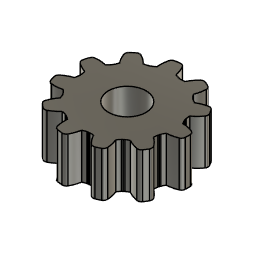
Pinion v6 (Autodesk Fusion 360 design; units mm, degrees)
Autodesk Fusion 360 part; units mm, degrees
(part 1 of 2)
sketch "Sketch1" plane through (0, 0, 0) normal (0, 0, 1) x (1, 0, 0)
sketch "Sketch2" plane through (0, 0, 0) normal (0, 0, 1) x (1, 0, 0)
  circle A0 centre (-2.1465, 3.0724) radius 9.2859
  spline S0 degree 5 poles (-1.9793, 9.7968) (-1.9628, 9.789) (-1.9296, 9.7738) (-1.8797, 9.7518) (-1.813, 9.7244) (-1.7292, 9.6933) (-1.6451, 9.6655) (-1.5605, 9.6411) (-1.4754, 9.6201) (-1.3897, 9.6025) (-1.3033, 9.5881) (-1.2161, 9.5769) (-1.128, 9.5685) (-1.039, 9.563) (-0.949, 9.5599) (-0.8581, 9.5593) (-0.7846, 9.5607) (-0.7291, 9.5627) (-0.6919, 9.5645) (-0.6732, 9.5655) knots 0 0 0 0 0 0 0.066667 0.133333 0.2 0.266667 0.333333 0.4 0.466667 0.533333 0.6 0.666667 0.733333 0.8 0.866667 0.933333 1 1 1 1 1 1
  line L0 (-2.6468, 6.3471) -> (-2.1465, 3.0724)
  spline S1 degree 5 poles (-4.3138, 9.4402) (-4.3273, 9.4278) (-4.3544, 9.4033) (-4.3954, 9.3675) (-4.4509, 9.3214) (-4.5216, 9.2667) (-4.5936, 9.2151) (-4.6671, 9.1665) (-4.742, 9.1211) (-4.8185, 9.0787) (-4.8967, 9.0392) (-4.9765, 9.0024) (-5.0581, 8.9682) (-5.1414, 8.9362) (-5.2264, 8.9065) (-5.313, 8.8788) (-5.3835, 8.8581) (-5.4371, 8.8435) (-5.4732, 8.8341) (-5.4913, 8.8295) knots 0 0 0 0 0 0 0.066667 0.133333 0.2 0.266667 0.333333 0.4 0.466667 0.533333 0.6 0.666667 0.733333 0.8 0.866667 0.933333 1 1 1 1 1 1
  line L1 (-2.1078, 9.8571) -> (-1.8509, 9.7365)
  line L2 (-0.8154, 9.5579) -> (-0.5311, 9.5732)
  line L3 (-4.2092, 9.5361) -> (-4.4184, 9.3442)
  line L4 (-5.3533, 8.8646) -> (-5.6292, 8.7944)
  arc A1 (-1.9793, 9.7968) -> (-3.3455, 12.2806) centre (-6.5618, 8.894) ccw
  arc A2 (-3.7515, 12.2186) -> (-4.3138, 9.4402) centre (0.3292, 9.9467) ccw
  arc A3 (-8.4415, 9.8989) -> (-7.4124, 7.2576) centre (-3.7804, 10.1939) ccw
  arc A4 (-5.6414, 8.8197) -> (-8.1335, 10.1706) centre (-9.0082, 5.5828) ccw
  spline S2 degree 5 poles (-5.6414, 8.8197) (-5.6232, 8.8221) (-5.587, 8.8272) (-5.5332, 8.8357) (-5.4623, 8.8487) (-5.375, 8.8679) (-5.2892, 8.89) (-5.2048, 8.9152) (-5.1219, 8.9435) (-5.0403, 8.9751) (-4.9598, 9.0097) (-4.8804, 9.0473) (-4.8018, 9.0879) (-4.7239, 9.1314) (-4.6466, 9.1775) (-4.5697, 9.2261) (-4.5086, 9.267) (-4.463, 9.2987) (-4.4327, 9.3204) (-4.4176, 9.3313) knots 0 0 0 0 0 0 0.066667 0.133333 0.2 0.266667 0.333333 0.4 0.466667 0.533333 0.6 0.666667 0.733333 0.8 0.866667 0.933333 1 1 1 1 1 1
  spline S3 degree 5 poles (-7.4124, 7.2576) (-7.4171, 7.2399) (-7.4267, 7.2046) (-7.4418, 7.1523) (-7.4636, 7.0835) (-7.4935, 6.9993) (-7.5261, 6.9169) (-7.5617, 6.8364) (-7.6001, 6.7576) (-7.6416, 6.6806) (-7.686, 6.6051) (-7.7333, 6.531) (-7.7834, 6.4581) (-7.8362, 6.3862) (-7.8916, 6.3153) (-7.9495, 6.2451) (-7.9977, 6.1896) (-8.0348, 6.1483) (-8.0601, 6.1209) (-8.0728, 6.1073) knots 0 0 0 0 0 0 0.066667 0.133333 0.2 0.266667 0.333333 0.4 0.466667 0.533333 0.6 0.666667 0.733333 0.8 0.866667 0.933333 1 1 1 1 1 1
  arc A5 (-11.1329, 5.4119) -> (-8.8391, 3.7463) centre (-7.3712, 8.1801) ccw
  arc A6 (-8.1938, 6.0179) -> (-11.0207, 5.807) centre (-9.2762, 1.4745) ccw
  spline S4 degree 5 poles (-8.1938, 6.0179) (-8.1798, 6.0297) (-8.1522, 6.0536) (-8.1115, 6.0898) (-8.0588, 6.1391) (-7.9958, 6.2024) (-7.9355, 6.2674) (-7.8782, 6.3342) (-7.8237, 6.4029) (-7.7721, 6.4735) (-7.7232, 6.5462) (-7.6767, 6.6208) (-7.6325, 6.6975) (-7.5905, 6.7761) (-7.5503, 6.8567) (-7.512, 6.9392) (-7.4827, 7.0066) (-7.4615, 7.0579) (-7.4477, 7.0925) (-7.4409, 7.1099) knots 0 0 0 0 0 0 0.066667 0.133333 0.2 0.266667 0.333333 0.4 0.466667 0.533333 0.6 0.666667 0.733333 0.8 0.866667 0.933333 1 1 1 1 1 1
  spline S5 degree 5 poles (-8.8391, 3.7463) (-8.8335, 3.7288) (-8.8225, 3.694) (-8.807, 3.6418) (-8.7881, 3.5722) (-8.7677, 3.4852) (-8.7506, 3.3982) (-8.737, 3.3112) (-8.7268, 3.2242) (-8.72, 3.137) (-8.7166, 3.0494) (-8.7163, 2.9615) (-8.719, 2.8731) (-8.7246, 2.7841) (-8.7328, 2.6944) (-8.7436, 2.6041) (-8.7541, 2.5314) (-8.7631, 2.4766) (-8.7695, 2.4399) (-8.7728, 2.4215) knots 0 0 0 0 0 0 0.066667 0.133333 0.2 0.266667 0.333333 0.4 0.466667 0.533333 0.6 0.666667 0.733333 0.8 0.866667 0.933333 1 1 1 1 1 1
  arc A7 (-10.9712, 0.1821) -> (-8.141, 0.021) centre (-9.3032, 4.5446) ccw
  arc A8 (-8.8263, 2.2809) -> (-11.0904, 0.5752) centre (-7.2805, -2.1264) ccw
  spline S6 degree 5 poles (-8.8263, 2.2809) (-8.8209, 2.2984) (-8.8105, 2.3334) (-8.7959, 2.3859) (-8.7783, 2.4559) (-8.7594, 2.5432) (-8.7439, 2.6305) (-8.7318, 2.7177) (-8.7231, 2.8049) (-8.7179, 2.8922) (-8.716, 2.9798) (-8.7172, 3.0677) (-8.7215, 3.156) (-8.7286, 3.2449) (-8.7384, 3.3344) (-8.7508, 3.4245) (-8.7626, 3.4971) (-8.7725, 3.5517) (-8.7796, 3.5883) (-8.7832, 3.6066) knots 0 0 0 0 0 0 0.066667 0.133333 0.2 0.266667 0.333333 0.4 0.466667 0.533333 0.6 0.666667 0.733333 0.8 0.866667 0.933333 1 1 1 1 1 1
  spline S7 degree 5 poles (-8.141, 0.021) (-8.1269, 0.0094) (-8.0988, -0.014) (-8.0575, -0.0495) (-8.004, -0.0979) (-7.9398, -0.16) (-7.8784, -0.224) (-7.8199, -0.2898) (-7.7643, -0.3575) (-7.7114, -0.4272) (-7.6612, -0.4989) (-7.6134, -0.5727) (-7.5679, -0.6486) (-7.5245, -0.7265) (-7.4829, -0.8064) (-7.4432, -0.8882) (-7.4127, -0.9551) (-7.3906, -1.006) (-7.3762, -1.0404) (-7.369, -1.0576) knots 0 0 0 0 0 0 0.066667 0.133333 0.2 0.266667 0.333333 0.4 0.466667 0.533333 0.6 0.666667 0.733333 0.8 0.866667 0.933333 1 1 1 1 1 1
  arc A9 (-8.0077, -4.1301) -> (-5.5397, -2.7355) centre (-8.963, 0.4417) ccw
  arc A10 (-7.338, -1.2048) -> (-8.3205, -3.8638) centre (-3.6548, -4.0767) ccw
  spline S8 degree 5 poles (-7.338, -1.2048) (-7.3429, -1.1872) (-7.3531, -1.1521) (-7.3692, -1.1) (-7.3922, -1.0316) (-7.4235, -0.948) (-7.4576, -0.8662) (-7.4946, -0.7863) (-7.5345, -0.7082) (-7.5773, -0.6319) (-7.623, -0.5572) (-7.6716, -0.484) (-7.723, -0.4119) (-7.777, -0.341) (-7.8337, -0.271) (-7.8928, -0.2019) (-7.9419, -0.1473) (-7.9798, -0.1066) (-8.0055, -0.0797) (-8.0185, -0.0663) knots 0 0 0 0 0 0 0.066667 0.133333 0.2 0.266667 0.333333 0.4 0.466667 0.533333 0.6 0.666667 0.733333 0.8 0.866667 0.933333 1 1 1 1 1 1
  spline S9 degree 5 poles (-5.5397, -2.7355) (-5.5215, -2.7376) (-5.4853, -2.7421) (-5.4313, -2.7496) (-5.3601, -2.7614) (-5.2725, -2.779) (-5.1863, -2.7996) (-5.1015, -2.8233) (-5.0181, -2.8502) (-4.936, -2.8803) (-4.8549, -2.9135) (-4.7749, -2.9497) (-4.6955, -2.9889) (-4.6169, -3.031) (-4.5388, -3.0757) (-4.4611, -3.123) (-4.3993, -3.1628) (-4.3531, -3.1937) (-4.3224, -3.2148) (-4.3071, -3.2255) knots 0 0 0 0 0 0 0.066667 0.133333 0.2 0.266667 0.333333 0.4 0.466667 0.533333 0.6 0.666667 0.733333 0.8 0.866667 0.933333 1 1 1 1 1 1
  arc A11 (-3.1833, -6.1555) -> (-1.8611, -3.648) centre (-6.4587, -2.826) ccw
  arc A12 (-4.2014, -3.3325) -> (-3.5904, -6.1006) centre (0.4497, -3.7573) ccw
  spline S10 degree 5 poles (-4.2014, -3.3325) (-4.2151, -3.3204) (-4.2427, -3.2964) (-4.2843, -3.2613) (-4.3406, -3.2162) (-4.4122, -3.1627) (-4.4852, -3.1124) (-4.5594, -3.0651) (-4.6352, -3.021) (-4.7124, -2.98) (-4.7913, -2.9419) (-4.8718, -2.9065) (-4.9539, -2.8737) (-5.0378, -2.8432) (-5.1233, -2.815) (-5.2103, -2.7888) (-5.2812, -2.7694) (-5.3351, -2.7557) (-5.3713, -2.7469) (-5.3895, -2.7427) knots 0 0 0 0 0 0 0.066667 0.133333 0.2 0.266667 0.333333 0.4 0.466667 0.533333 0.6 0.666667 0.733333 0.8 0.866667 0.933333 1 1 1 1 1 1
  spline S11 degree 5 poles (-1.8611, -3.648) (-1.8446, -3.6399) (-1.8117, -3.6241) (-1.7622, -3.6013) (-1.696, -3.5727) (-1.6128, -3.5401) (-1.5292, -3.5109) (-1.445, -3.485) (-1.3603, -3.4625) (-1.2749, -3.4434) (-1.1888, -3.4275) (-1.1018, -3.4147) (-1.0139, -3.4048) (-0.925, -3.3977) (-0.8351, -3.3931) (-0.7442, -3.3909) (-0.6707, -3.3909) (-0.6151, -3.392) (-0.5779, -3.3931) (-0.5592, -3.3938) knots 0 0 0 0 0 0 0.066667 0.133333 0.2 0.266667 0.333333 0.4 0.466667 0.533333 0.6 0.666667 0.733333 0.8 0.866667 0.933333 1 1 1 1 1 1
  arc A13 (1.9703, -5.2511) -> (1.727, -2.4268) centre (-2.5852, -4.2209) ccw
  arc A14 (-0.4125, -3.4267) -> (1.5981, -5.425) centre (3.73, -1.2694) ccw
  spline S12 degree 5 poles (-0.4125, -3.4267) (-0.4306, -3.4239) (-0.4667, -3.4186) (-0.5207, -3.4116) (-0.5925, -3.4041) (-0.6816, -3.3979) (-0.7702, -3.3949) (-0.8582, -3.3953) (-0.9458, -3.3992) (-1.033, -3.4064) (-1.1199, -3.417) (-1.2067, -3.4307) (-1.2936, -3.4476) (-1.3806, -3.4673) (-1.4678, -3.4897) (-1.5552, -3.5148) (-1.6253, -3.5368) (-1.678, -3.5544) (-1.7132, -3.5666) (-1.7308, -3.5728) knots 0 0 0 0 0 0 0.066667 0.133333 0.2 0.266667 0.333333 0.4 0.466667 0.533333 0.6 0.666667 0.733333 0.8 0.866667 0.933333 1 1 1 1 1 1
  spline S13 degree 5 poles (1.727, -2.4268) (1.7364, -2.4112) (1.7555, -2.38) (1.7848, -2.3341) (1.8251, -2.2742) (1.8775, -2.2019) (1.932, -2.132) (1.9888, -2.0647) (2.0479, -2) (2.1094, -1.9378) (2.1733, -1.8779) (2.2395, -1.8201) (2.3082, -1.7642) (2.3791, -1.7102) (2.4522, -1.6577) (2.5275, -1.6067) (2.5894, -1.567) (2.6367, -1.5379) (2.6686, -1.5187) (2.6847, -1.5092) knots 0 0 0 0 0 0 0.066667 0.133333 0.2 0.266667 0.333333 0.4 0.466667 0.533333 0.6 0.666667 0.733333 0.8 0.866667 0.933333 1 1 1 1 1 1
  arc A15 (5.8168, -1.7041) -> (4.0852, 0.5403) centre (1.4275, -3.3003) ccw
  arc A16 (2.8259, -1.4575) -> (5.5977, -2.0516) centre (5.1445, 2.5969) ccw
  spline S14 degree 5 poles (2.8259, -1.4575) (2.8092, -1.4649) (2.776, -1.48) (2.7267, -1.5033) (2.6623, -1.5358) (2.5839, -1.5787) (2.5078, -1.6241) (2.434, -1.6721) (2.3624, -1.7227) (2.293, -1.7759) (2.2256, -1.8318) (2.1599, -1.8903) (2.096, -1.9514) (2.0334, -2.015) (1.9722, -2.081) (1.9122, -2.1494) (1.8651, -2.2058) (1.8303, -2.2491) (1.8073, -2.2784) (1.7959, -2.2931) knots 0 0 0 0 0 0 0.066667 0.133333 0.2 0.266667 0.333333 0.4 0.466667 0.533333 0.6 0.666667 0.733333 0.8 0.866667 0.933333 1 1 1 1 1 1
  spline S15 degree 5 poles (4.0852, 0.5403) (4.0846, 0.5586) (4.0839, 0.5951) (4.0837, 0.6496) (4.0852, 0.7217) (4.0902, 0.8109) (4.0983, 0.8992) (4.1097, 0.9865) (4.1244, 1.0729) (4.1425, 1.1585) (4.1639, 1.2434) (4.1883, 1.3279) (4.2159, 1.4119) (4.2463, 1.4958) (4.2795, 1.5795) (4.3152, 1.6631) (4.3458, 1.7299) (4.3699, 1.78) (4.3864, 1.8134) (4.3947, 1.8301) knots 0 0 0 0 0 0 0.066667 0.133333 0.2 0.266667 0.333333 0.4 0.466667 0.533333 0.6 0.666667 0.733333 0.8 0.866667 0.933333 1 1 1 1 1 1
  arc A17 (7.135, 3.3594) -> (4.4649, 4.3114) centre (4.3055, -0.3564) ccw
  arc A18 (4.4856, 1.9499) -> (7.1386, 2.9487) centre (4.2442, 6.6142) ccw
  spline S16 degree 5 poles (4.4856, 1.9499) (4.4756, 1.9346) (4.4557, 1.904) (4.4269, 1.8577) (4.3903, 1.7956) (4.3476, 1.7171) (4.3081, 1.6378) (4.2719, 1.5575) (4.239, 1.4762) (4.2094, 1.3939) (4.1829, 1.3105) (4.1593, 1.2258) (4.1386, 1.1398) (4.1204, 1.0525) (4.1046, 0.9638) (4.091, 0.8739) (4.0819, 0.801) (4.076, 0.7457) (4.0725, 0.7086) (4.0709, 0.69) knots 0 0 0 0 0 0 0.066667 0.133333 0.2 0.266667 0.333333 0.4 0.466667 0.533333 0.6 0.666667 0.733333 0.8 0.866667 0.933333 1 1 1 1 1 1
  spline S17 degree 5 poles (4.4649, 4.3114) (4.4545, 4.3265) (4.4342, 4.3568) (4.4045, 4.4026) (4.3668, 4.464) (4.3228, 4.5418) (4.2819, 4.6204) (4.2443, 4.7) (4.21, 4.7806) (4.1789, 4.8624) (4.1509, 4.9454) (4.1259, 5.0297) (4.1036, 5.1153) (4.0838, 5.2023) (4.0665, 5.2906) (4.0514, 5.3803) (4.041, 5.4531) (4.0341, 5.5082) (4.03, 5.5452) (4.028, 5.5638) knots 0 0 0 0 0 0 0.066667 0.133333 0.2 0.266667 0.333333 0.4 0.466667 0.533333 0.6 0.666667 0.733333 0.8 0.866667 0.933333 1 1 1 1 1 1
  arc A19 (5.5064, 8.3318) -> (2.7455, 7.6891) centre (5.135, 3.6761) ccw
  arc A20 (4.0396, 5.7137) -> (5.7315, 7.9882) centre (1.3148, 9.507) ccw
  spline S18 degree 5 poles (4.0396, 5.7137) (4.0395, 5.6954) (4.0394, 5.6589) (4.0401, 5.6044) (4.0429, 5.5323) (4.0494, 5.4432) (4.0591, 5.3551) (4.072, 5.268) (4.0883, 5.1819) (4.1079, 5.0967) (4.1307, 5.0121) (4.1567, 4.9281) (4.1857, 4.8445) (4.2176, 4.7612) (4.2522, 4.6781) (4.2894, 4.5952) (4.3212, 4.5289) (4.3461, 4.4792) (4.3632, 4.4461) (4.3719, 4.4296) knots 0 0 0 0 0 0 0.066667 0.133333 0.2 0.266667 0.333333 0.4 0.466667 0.533333 0.6 0.666667 0.733333 0.8 0.866667 0.933333 1 1 1 1 1 1
  spline S19 degree 5 poles (2.7455, 7.6891) (2.7286, 7.6962) (2.6951, 7.7107) (2.6454, 7.7332) (2.5805, 7.7645) (2.5014, 7.8061) (2.4245, 7.8501) (2.3498, 7.8967) (2.2773, 7.946) (2.207, 7.998) (2.1386, 8.0527) (2.072, 8.1101) (2.0069, 8.1701) (1.9433, 8.2326) (1.8809, 8.2975) (1.8197, 8.3648) (1.7717, 8.4204) (1.7361, 8.463) (1.7126, 8.4919) (1.7009, 8.5065) knots 0 0 0 0 0 0 0.066667 0.133333 0.2 0.266667 0.333333 0.4 0.466667 0.533333 0.6 0.666667 0.733333 0.8 0.866667 0.933333 1 1 1 1 1 1
  arc A21 (1.4481, 11.6344) -> (-0.5271, 9.601) centre (3.6527, 7.517) ccw
  arc A22 (1.6296, 8.6389) -> (1.8232, 11.467) centre (-2.7135, 10.3569) ccw
  spline S20 degree 5 poles (1.6296, 8.6389) (1.6393, 8.6234) (1.659, 8.5926) (1.6891, 8.5472) (1.7304, 8.4881) (1.7841, 8.4166) (1.8398, 8.3478) (1.8978, 8.2815) (1.958, 8.2178) (2.0206, 8.1567) (2.0855, 8.0979) (2.1528, 8.0413) (2.2224, 7.9867) (2.2942, 7.9338) (2.3683, 7.8826) (2.4445, 7.833) (2.507, 7.7944) (2.5548, 7.7661) (2.5871, 7.7475) (2.6033, 7.7383) knots 0 0 0 0 0 0 0.066667 0.133333 0.2 0.266667 0.333333 0.4 0.466667 0.533333 0.6 0.666667 0.733333 0.8 0.866667 0.933333 1 1 1 1 1 1
  spline S21 degree 5 poles (-0.5271, 9.601) (-0.5451, 9.5979) (-0.5812, 9.592) (-0.6351, 9.584) (-0.7067, 9.5752) (-0.7957, 9.5674) (-0.8842, 9.5629) (-0.9722, 9.5618) (-1.0598, 9.5641) (-1.1471, 9.5698) (-1.2342, 9.5788) (-1.3213, 9.5911) (-1.4084, 9.6063) (-1.4957, 9.6245) (-1.5833, 9.6454) (-1.6712, 9.669) (-1.7417, 9.6897) (-1.7947, 9.7064) (-1.8301, 9.718) (-1.8478, 9.7239) knots 0 0 0 0 0 0 0.066667 0.133333 0.2 0.266667 0.333333 0.4 0.466667 0.533333 0.6 0.666667 0.733333 0.8 0.866667 0.933333 1 1 1 1 1 1
  point P0 (-1.5603, 9.642)
  point P1 (-1.1296, 9.5694)
  point P2 (-4.6674, 9.1673)
  point P3 (-5.0568, 8.9694)
  point P4 (-5.2052, 8.916)
  point P5 (-4.8036, 9.0878)
  point P6 (-7.5624, 6.8368)
  point P7 (-7.783, 6.4599)
  point P8 (-7.8789, 6.3347)
  point P9 (-7.6339, 6.6963)
  point P10 (-8.7378, 3.3112)
  point P11 (-8.7196, 2.8748)
  point P12 (-8.7326, 2.7177)
  point P13 (-8.7221, 3.1543)
  point P14 (-7.8206, -0.2903)
  point P15 (-7.5693, -0.6475)
  point P16 (-7.4953, -0.7867)
  point P17 (-7.7225, -0.4137)
  point P18 (-5.1019, -2.8241)
  point P19 (-4.6973, -2.9888)
  point P20 (-4.5598, -3.0659)
  point P21 (-4.9526, -2.8749)
  point P22 (-1.4448, -3.4858)
  point P23 (-1.0155, -3.4057)
  point P24 (-0.8581, -3.3962)
  point P25 (-1.2918, -3.4479)
  point P26 (1.9894, -2.0654)
  point P27 (2.3073, -1.7658)
  point P28 (2.4345, -1.6728)
  point P29 (2.0976, -1.9507)
  point P30 (4.1105, 0.9863)
  point P31 (4.216, 1.4101)
  point P32 (4.2727, 1.5572)
  point P33 (4.1396, 1.1412)
  point P34 (4.2451, 4.7003)
  point P35 (4.1047, 5.1139)
  point P36 (4.0729, 5.2683)
  point P37 (4.1858, 4.8463)
  point P38 (2.3504, 7.8974)
  point P39 (2.0086, 8.1694)
  point P40 (1.8984, 8.2821)
  point P41 (2.2215, 7.9882)
  point P42 (-0.9721, 9.5627)
  point P43 (-1.4067, 9.6067)
  dimension "d2" = 360
  constraint coincident A0.centre L0.end
  constraint midpoint S0.start L1
  constraint midpoint S0.end L2
  constraint symmetric S0.start L0 S1.start
  constraint symmetric P0 L0 P2
  constraint symmetric P1 L0 P3
  constraint symmetric S0.end L0 S1.end
  constraint symmetric L0 L1.start L3.start
  constraint symmetric L0 L1.end L3.end
  constraint symmetric L0 L2.start L4.start
  constraint symmetric L0 L2.end L4.end
  constraint coincident A0 A1.end
  constraint coincident A0 A2.start
  constraint coincident L0.start A2
extrude "Extrude1" add sketch "Sketch2" along normal blind 6.35 contours A0 S0 S1 A1 A2 A3 A4 S2 S3 A5 A6 S4 S5 A7 A8 S6 S7 A9 A10 S8 S9 A11 A12 S10 S11 A13 A14 S12 S13 A15 A16 S14 S15 A17 A18 S16 S17 A19 A20 S18 S19 A21 A22 S20 S21
sketch "Sketch3" plane through (0, 0, 6.35) normal (0, 0, 1) x (-1, 0, 0)
  arc A0 (-1.6296, -8.6389) -> (-1.8232, -11.467) centre (2.7135, -10.3569) ccw
  arc A1 (-1.8232, -11.467) -> (-1.4481, -11.6344) centre (2.1465, -3.0724) ccw
  arc A2 (-1.4481, -11.6344) -> (0.5271, -9.601) centre (-3.6527, -7.517) ccw
  spline S0 degree 5 poles (0.5271, -9.601) (0.5451, -9.5979) (0.5812, -9.592) (0.6351, -9.584) (0.7067, -9.5752) (0.7957, -9.5674) (0.8842, -9.5629) (0.9616, -9.5619) (1.0213, -9.5631) (1.0633, -9.565) (1.0877, -9.5664) (1.0947, -9.5668) knots 0 0 0 0 0 0 0.066667 0.133333 0.2 0.266667 0.333333 0.4 0.426673 0.426673 0.426673 0.426673 0.426673 0.426673
  spline S1 degree 5 poles (1.0947, -9.5668) (1.1052, -9.5675) (1.1331, -9.5693) (1.1679, -9.5722) (1.2027, -9.5757) (1.2375, -9.5799) (1.2618, -9.5831) (1.2687, -9.5841) knots 0.426673 0.426673 0.426673 0.426673 0.426673 0.426673 0.466667 0.533333 0.559717 0.559717 0.559717 0.559717 0.559717 0.559717
  spline S2 degree 5 poles (1.2687, -9.5841) (1.2756, -9.585) (1.2999, -9.5883) (1.3345, -9.5935) (1.369, -9.5993) (1.4033, -9.6058) (1.4307, -9.6113) (1.441, -9.6135) knots -0.559717 -0.559717 -0.559717 -0.559717 -0.559717 -0.559717 -0.533333 -0.466667 -0.426673 -0.426673 -0.426673 -0.426673 -0.426673 -0.426673
  spline S3 degree 5 poles (1.441, -9.6135) (1.4479, -9.6149) (1.4718, -9.6201) (1.5128, -9.6294) (1.5706, -9.644) (1.6451, -9.6655) (1.7292, -9.6933) (1.813, -9.7244) (1.8797, -9.7518) (1.9296, -9.7738) (1.9628, -9.789) (1.9793, -9.7968) knots -0.426673 -0.426673 -0.426673 -0.426673 -0.426673 -0.426673 -0.4 -0.333333 -0.266667 -0.2 -0.133333 -0.066667 0 0 0 0 0 0
  arc A3 (1.9793, -9.7968) -> (3.3455, -12.2806) centre (6.5618, -8.894) ccw
  arc A4 (3.3455, -12.2806) -> (3.7515, -12.2186) centre (2.1465, -3.0724) ccw
  arc A5 (3.7515, -12.2186) -> (4.3138, -9.4402) centre (-0.3292, -9.9467) ccw
  spline S4 degree 5 poles (4.3138, -9.4402) (4.3273, -9.4278) (4.3544, -9.4033) (4.3954, -9.3675) (4.4509, -9.3214) (4.5216, -9.2667) (4.5936, -9.2151) (4.6582, -9.1723) (4.7091, -9.1411) (4.7454, -9.12) (4.7667, -9.1079) (4.7728, -9.1045) knots 0 0 0 0 0 0 0.066667 0.133333 0.2 0.266667 0.333333 0.4 0.426673 0.426673 0.426673 0.426673 0.426673 0.426673
  spline S5 degree 5 poles (4.7728, -9.1045) (4.782, -9.0994) (4.8065, -9.0859) (4.8373, -9.0695) (4.8685, -9.0536) (4.9, -9.0383) (4.9222, -9.0279) (4.9285, -9.025) knots 0.426673 0.426673 0.426673 0.426673 0.426673 0.426673 0.466667 0.533333 0.559717 0.559717 0.559717 0.559717 0.559717 0.559717
  spline S6 degree 5 poles (4.9285, -9.025) (4.9348, -9.022) (4.9571, -9.0117) (4.989, -8.9973) (5.0211, -8.9836) (5.0535, -8.9704) (5.0796, -8.9603) (5.0894, -8.9566) knots -0.559717 -0.559717 -0.559717 -0.559717 -0.559717 -0.559717 -0.533333 -0.466667 -0.426673 -0.426673 -0.426673 -0.426673 -0.426673 -0.426673
  spline S7 degree 5 poles (5.0894, -8.9566) (5.0959, -8.9541) (5.1189, -8.9454) (5.1584, -8.9311) (5.2149, -8.9122) (5.2892, -8.89) (5.375, -8.8679) (5.4623, -8.8487) (5.5332, -8.8357) (5.587, -8.8272) (5.6232, -8.8221) (5.6414, -8.8197) knots -0.426673 -0.426673 -0.426673 -0.426673 -0.426673 -0.426673 -0.4 -0.333333 -0.266667 -0.2 -0.133333 -0.066667 0 0 0 0 0 0
  arc A6 (5.6414, -8.8197) -> (8.1335, -10.1706) centre (9.0082, -5.5828) ccw
  arc A7 (8.1335, -10.1706) -> (8.4415, -9.8989) centre (2.1465, -3.0724) ccw
  arc A8 (8.4415, -9.8989) -> (7.4124, -7.2576) centre (3.7804, -10.1939) ccw
  spline S8 degree 5 poles (7.4124, -7.2576) (7.4171, -7.2399) (7.4267, -7.2046) (7.4418, -7.1523) (7.4636, -7.0835) (7.4935, -6.9993) (7.5261, -6.9169) (7.5574, -6.8461) (7.5833, -6.7923) (7.6024, -6.7549) (7.6138, -6.7332) (7.6171, -6.727) knots 0 0 0 0 0 0 0.066667 0.133333 0.2 0.266667 0.333333 0.4 0.426673 0.426673 0.426673 0.426673 0.426673 0.426673
  spline S9 degree 5 poles (7.6171, -6.727) (7.6221, -6.7178) (7.6354, -6.6931) (7.6524, -6.6627) (7.6701, -6.6325) (7.6883, -6.6026) (7.7014, -6.5818) (7.7051, -6.576) knots 0.426673 0.426673 0.426673 0.426673 0.426673 0.426673 0.466667 0.533333 0.559717 0.559717 0.559717 0.559717 0.559717 0.559717
  spline S10 degree 5 poles (7.7051, -6.576) (7.7088, -6.5701) (7.7219, -6.5494) (7.741, -6.52) (7.7606, -6.4911) (7.7807, -6.4625) (7.7972, -6.4399) (7.8034, -6.4314) knots -0.559717 -0.559717 -0.559717 -0.559717 -0.559717 -0.559717 -0.533333 -0.466667 -0.426673 -0.426673 -0.426673 -0.426673 -0.426673 -0.426673
  spline S11 degree 5 poles (7.8034, -6.4314) (7.8076, -6.4258) (7.8222, -6.4061) (7.8477, -6.3727) (7.885, -6.3262) (7.9355, -6.2674) (7.9958, -6.2024) (8.0588, -6.1391) (8.1115, -6.0898) (8.1522, -6.0536) (8.1798, -6.0297) (8.1938, -6.0179) knots -0.426673 -0.426673 -0.426673 -0.426673 -0.426673 -0.426673 -0.4 -0.333333 -0.266667 -0.2 -0.133333 -0.066667 0 0 0 0 0 0
  arc A9 (8.1938, -6.0179) -> (11.0207, -5.807) centre (9.2762, -1.4745) ccw
  arc A10 (11.0207, -5.807) -> (11.1329, -5.4119) centre (2.1465, -3.0724) ccw
  arc A11 (11.1329, -5.4119) -> (8.8391, -3.7463) centre (7.3712, -8.1801) ccw
  spline S12 degree 5 poles (8.8391, -3.7463) (8.8335, -3.7288) (8.8225, -3.694) (8.807, -3.6418) (8.7881, -3.5722) (8.7677, -3.4852) (8.7506, -3.3982) (8.7386, -3.3217) (8.7313, -3.2625) (8.7272, -3.2207) (8.7251, -3.1962) (8.7245, -3.1893) knots 0 0 0 0 0 0 0.066667 0.133333 0.2 0.266667 0.333333 0.4 0.426673 0.426673 0.426673 0.426673 0.426673 0.426673
  spline S13 degree 5 poles (8.7245, -3.1893) (8.7237, -3.1788) (8.7216, -3.1509) (8.7194, -3.116) (8.718, -3.0811) (8.7172, -3.0461) (8.7169, -3.0216) (8.7169, -3.0146) knots 0.426673 0.426673 0.426673 0.426673 0.426673 0.426673 0.466667 0.533333 0.559717 0.559717 0.559717 0.559717 0.559717 0.559717
  spline S14 degree 5 poles (8.7169, -3.0146) (8.7168, -3.0076) (8.7166, -2.9831) (8.7168, -2.9481) (8.7177, -2.9132) (8.7192, -2.8783) (8.7208, -2.8503) (8.7215, -2.8398) knots -0.559717 -0.559717 -0.559717 -0.559717 -0.559717 -0.559717 -0.533333 -0.466667 -0.426673 -0.426673 -0.426673 -0.426673 -0.426673 -0.426673
  spline S15 degree 5 poles (8.7215, -2.8398) (8.7219, -2.8328) (8.7236, -2.8084) (8.727, -2.7665) (8.7332, -2.7072) (8.7439, -2.6305) (8.7594, -2.5432) (8.7783, -2.4559) (8.7959, -2.3859) (8.8105, -2.3334) (8.8209, -2.2984) (8.8263, -2.2809) knots -0.426673 -0.426673 -0.426673 -0.426673 -0.426673 -0.426673 -0.4 -0.333333 -0.266667 -0.2 -0.133333 -0.066667 0 0 0 0 0 0
  arc A12 (8.8263, -2.2809) -> (11.0904, -0.5752) centre (7.2805, 2.1264) ccw
  arc A13 (11.0904, -0.5752) -> (10.9712, -0.1821) centre (2.1465, -3.0724) ccw
  arc A14 (10.9712, -0.1821) -> (8.141, -0.021) centre (9.3032, -4.5446) ccw
  spline S16 degree 5 poles (8.141, -0.021) (8.1269, -0.0094) (8.0988, 0.014) (8.0575, 0.0495) (8.004, 0.0979) (7.9398, 0.16) (7.8784, 0.224) (7.8269, 0.2819) (7.7888, 0.3277) (7.7627, 0.3607) (7.7477, 0.3801) (7.7435, 0.3856) knots 0 0 0 0 0 0 0.066667 0.133333 0.2 0.266667 0.333333 0.4 0.426673 0.426673 0.426673 0.426673 0.426673 0.426673
  spline S17 degree 5 poles (7.7435, 0.3856) (7.7371, 0.394) (7.7202, 0.4163) (7.6996, 0.4445) (7.6795, 0.4731) (7.6599, 0.5021) (7.6464, 0.5226) (7.6426, 0.5284) knots 0.426673 0.426673 0.426673 0.426673 0.426673 0.426673 0.466667 0.533333 0.559717 0.559717 0.559717 0.559717 0.559717 0.559717
  spline S18 degree 5 poles (7.6426, 0.5284) (7.6388, 0.5342) (7.6254, 0.5548) (7.6066, 0.5843) (7.5884, 0.6142) (7.5708, 0.6443) (7.5571, 0.6687) (7.552, 0.6779) knots -0.559717 -0.559717 -0.559717 -0.559717 -0.559717 -0.559717 -0.533333 -0.466667 -0.426673 -0.426673 -0.426673 -0.426673 -0.426673 -0.426673
  spline S19 degree 5 poles (7.552, 0.6779) (7.5486, 0.684) (7.5367, 0.7055) (7.517, 0.7426) (7.4902, 0.7959) (7.4576, 0.8662) (7.4235, 0.948) (7.3922, 1.0316) (7.3692, 1.1) (7.3531, 1.1521) (7.3429, 1.1872) (7.338, 1.2048) knots -0.426673 -0.426673 -0.426673 -0.426673 -0.426673 -0.426673 -0.4 -0.333333 -0.266667 -0.2 -0.133333 -0.066667 0 0 0 0 0 0
  arc A15 (7.338, 1.2048) -> (8.3205, 3.8638) centre (3.6548, 4.0767) ccw
  arc A16 (8.3205, 3.8638) -> (8.0077, 4.1301) centre (2.1465, -3.0724) ccw
  arc A17 (8.0077, 4.1301) -> (5.5397, 2.7355) centre (8.963, -0.4417) ccw
  spline S20 degree 5 poles (5.5397, 2.7355) (5.5215, 2.7376) (5.4853, 2.7421) (5.4313, 2.7496) (5.3601, 2.7614) (5.2725, 2.779) (5.1863, 2.7996) (5.1117, 2.8204) (5.0549, 2.8384) (5.0151, 2.852) (4.992, 2.8602) (4.9854, 2.8626) knots 0 0 0 0 0 0 0.066667 0.133333 0.2 0.266667 0.333333 0.4 0.426673 0.426673 0.426673 0.426673 0.426673 0.426673
  spline S21 degree 5 poles (4.9854, 2.8626) (4.9755, 2.8662) (4.9493, 2.8759) (4.9167, 2.8884) (4.8843, 2.9016) (4.8521, 2.9154) (4.8297, 2.9254) (4.8234, 2.9282) knots 0.426673 0.426673 0.426673 0.426673 0.426673 0.426673 0.466667 0.533333 0.559717 0.559717 0.559717 0.559717 0.559717 0.559717
  spline S22 degree 5 poles (4.8234, 2.9282) (4.817, 2.931) (4.7946, 2.9411) (4.7629, 2.9558) (4.7314, 2.9711) (4.7003, 2.9869) (4.6756, 3) (4.6663, 3.005) knots -0.559717 -0.559717 -0.559717 -0.559717 -0.559717 -0.559717 -0.533333 -0.466667 -0.426673 -0.426673 -0.426673 -0.426673 -0.426673 -0.426673
  spline S23 degree 5 poles (4.6663, 3.005) (4.6601, 3.0083) (4.6386, 3.02) (4.6019, 3.0405) (4.5505, 3.0708) (4.4852, 3.1124) (4.4122, 3.1627) (4.3406, 3.2162) (4.2843, 3.2613) (4.2427, 3.2964) (4.2151, 3.3204) (4.2014, 3.3325) knots -0.426673 -0.426673 -0.426673 -0.426673 -0.426673 -0.426673 -0.4 -0.333333 -0.266667 -0.2 -0.133333 -0.066667 0 0 0 0 0 0
  arc A18 (4.2014, 3.3325) -> (3.5904, 6.1006) centre (-0.4497, 3.7573) ccw
  arc A19 (3.5904, 6.1006) -> (3.1833, 6.1555) centre (2.1465, -3.0724) ccw
  arc A20 (3.1833, 6.1555) -> (1.8611, 3.648) centre (6.4587, 2.826) ccw
  spline S24 degree 5 poles (1.8611, 3.648) (1.8446, 3.6399) (1.8117, 3.6241) (1.7622, 3.6013) (1.696, 3.5727) (1.6128, 3.5401) (1.5292, 3.5109) (1.4551, 3.4881) (1.3975, 3.4724) (1.3567, 3.4624) (1.3329, 3.4568) (1.326, 3.4553) knots 0 0 0 0 0 0 0.066667 0.133333 0.2 0.266667 0.333333 0.4 0.426673 0.426673 0.426673 0.426673 0.426673 0.426673
  spline S25 degree 5 poles (1.326, 3.4553) (1.3158, 3.4529) (1.2885, 3.4469) (1.2543, 3.4398) (1.2199, 3.4334) (1.1854, 3.4276) (1.1611, 3.4239) (1.1543, 3.4228) knots 0.426673 0.426673 0.426673 0.426673 0.426673 0.426673 0.466667 0.533333 0.559717 0.559717 0.559717 0.559717 0.559717 0.559717
  spline S26 degree 5 poles (1.1543, 3.4228) (1.1474, 3.4218) (1.1231, 3.4181) (1.0884, 3.4133) (1.0537, 3.4092) (1.019, 3.4057) (0.9911, 3.4033) (0.9806, 3.4025) knots -0.559717 -0.559717 -0.559717 -0.559717 -0.559717 -0.559717 -0.533333 -0.466667 -0.426673 -0.426673 -0.426673 -0.426673 -0.426673 -0.426673
  spline S27 degree 5 poles (0.9806, 3.4025) (0.9736, 3.402) (0.9492, 3.4001) (0.9072, 3.3975) (0.8476, 3.3953) (0.7702, 3.3949) (0.6816, 3.3979) (0.5925, 3.4041) (0.5207, 3.4116) (0.4667, 3.4186) (0.4306, 3.4239) (0.4125, 3.4267) knots -0.426673 -0.426673 -0.426673 -0.426673 -0.426673 -0.426673 -0.4 -0.333333 -0.266667 -0.2 -0.133333 -0.066667 0 0 0 0 0 0
  arc A21 (0.4125, 3.4267) -> (-1.5981, 5.425) centre (-3.73, 1.2694) ccw
  arc A22 (-1.5981, 5.425) -> (-1.9703, 5.2511) centre (2.1465, -3.0724) ccw
  arc A23 (-1.9703, 5.2511) -> (-1.727, 2.4268) centre (2.5852, 4.2209) ccw
  spline S28 degree 5 poles (-1.727, 2.4268) (-1.7364, 2.4112) (-1.7555, 2.38) (-1.7848, 2.3341) (-1.8251, 2.2742) (-1.8775, 2.2019) (-1.932, 2.132) (-1.982, 2.0728) (-2.022, 2.0286) (-2.0509, 1.998) (-2.0679, 1.9805) (-2.0728, 1.9755) knots 0 0 0 0 0 0 0.066667 0.133333 0.2 0.266667 0.333333 0.4 0.426673 0.426673 0.426673 0.426673 0.426673 0.426673
  spline S29 degree 5 poles (-2.0728, 1.9755) (-2.0802, 1.968) (-2.0999, 1.9481) (-2.1249, 1.9236) (-2.1503, 1.8997) (-2.1762, 1.8761) (-2.1946, 1.8599) (-2.1998, 1.8553) knots 0.426673 0.426673 0.426673 0.426673 0.426673 0.426673 0.466667 0.533333 0.559717 0.559717 0.559717 0.559717 0.559717 0.559717
  spline S30 degree 5 poles (-2.1998, 1.8553) (-2.205, 1.8507) (-2.2235, 1.8345) (-2.25, 1.8117) (-2.277, 1.7895) (-2.3044, 1.7677) (-2.3265, 1.7507) (-2.3349, 1.7443) knots -0.559717 -0.559717 -0.559717 -0.559717 -0.559717 -0.559717 -0.533333 -0.466667 -0.426673 -0.426673 -0.426673 -0.426673 -0.426673 -0.426673
  spline S31 degree 5 poles (-2.3349, 1.7443) (-2.3405, 1.7401) (-2.36, 1.7253) (-2.3939, 1.7005) (-2.4429, 1.6663) (-2.5078, 1.6241) (-2.5839, 1.5787) (-2.6623, 1.5358) (-2.7267, 1.5033) (-2.776, 1.48) (-2.8092, 1.4649) (-2.8259, 1.4575) knots -0.426673 -0.426673 -0.426673 -0.426673 -0.426673 -0.426673 -0.4 -0.333333 -0.266667 -0.2 -0.133333 -0.066667 0 0 0 0 0 0
  arc A24 (-2.8259, 1.4575) -> (-5.5977, 2.0516) centre (-5.1445, -2.5969) ccw
  arc A25 (-5.5977, 2.0516) -> (-5.8168, 1.7041) centre (2.1465, -3.0724) ccw
  arc A26 (-5.8168, 1.7041) -> (-4.0852, -0.5403) centre (-1.4275, 3.3003) ccw
  spline S32 degree 5 poles (-4.0852, -0.5403) (-4.0846, -0.5586) (-4.0839, -0.5951) (-4.0837, -0.6496) (-4.0852, -0.7217) (-4.0902, -0.8109) (-4.0983, -0.8992) (-4.1083, -0.976) (-4.118, -1.0349) (-4.1258, -1.0762) (-4.1307, -1.1002) (-4.1321, -1.107) knots 0 0 0 0 0 0 0.066667 0.133333 0.2 0.266667 0.333333 0.4 0.426673 0.426673 0.426673 0.426673 0.426673 0.426673
  spline S33 degree 5 poles (-4.1321, -1.107) (-4.1342, -1.1173) (-4.1401, -1.1447) (-4.1479, -1.1788) (-4.1563, -1.2127) (-4.1654, -1.2465) (-4.172, -1.2701) (-4.174, -1.2768) knots 0.426673 0.426673 0.426673 0.426673 0.426673 0.426673 0.466667 0.533333 0.559717 0.559717 0.559717 0.559717 0.559717 0.559717
  spline S34 degree 5 poles (-4.174, -1.2768) (-4.1758, -1.2835) (-4.1826, -1.3071) (-4.1927, -1.3406) (-4.2033, -1.3739) (-4.2146, -1.4069) (-4.224, -1.4333) (-4.2276, -1.4432) knots -0.559717 -0.559717 -0.559717 -0.559717 -0.559717 -0.559717 -0.533333 -0.466667 -0.426673 -0.426673 -0.426673 -0.426673 -0.426673 -0.426673
  spline S35 degree 5 poles (-4.2276, -1.4432) (-4.23, -1.4498) (-4.2385, -1.4727) (-4.2536, -1.512) (-4.2763, -1.5671) (-4.3081, -1.6378) (-4.3476, -1.7171) (-4.3903, -1.7956) (-4.4269, -1.8577) (-4.4557, -1.904) (-4.4756, -1.9346) (-4.4856, -1.9499) knots -0.426673 -0.426673 -0.426673 -0.426673 -0.426673 -0.426673 -0.4 -0.333333 -0.266667 -0.2 -0.133333 -0.066667 0 0 0 0 0 0
  arc A27 (-4.4856, -1.9499) -> (-7.1386, -2.9487) centre (-4.2442, -6.6142) ccw
  arc A28 (-7.1386, -2.9487) -> (-7.135, -3.3594) centre (2.1465, -3.0724) ccw
  arc A29 (-7.135, -3.3594) -> (-4.4649, -4.3114) centre (-4.3055, 0.3564) ccw
  spline S36 degree 5 poles (-4.4649, -4.3114) (-4.4545, -4.3265) (-4.4342, -4.3568) (-4.4045, -4.4026) (-4.3668, -4.464) (-4.3228, -4.5418) (-4.2819, -4.6204) (-4.2488, -4.6904) (-4.2251, -4.7452) (-4.2093, -4.7841) (-4.2005, -4.807) (-4.198, -4.8135) knots 0 0 0 0 0 0 0.066667 0.133333 0.2 0.266667 0.333333 0.4 0.426673 0.426673 0.426673 0.426673 0.426673 0.426673
  spline S37 degree 5 poles (-4.198, -4.8135) (-4.1942, -4.8233) (-4.1843, -4.8495) (-4.1724, -4.8824) (-4.1612, -4.9155) (-4.1506, -4.9488) (-4.1434, -4.9723) (-4.1414, -4.9789) knots 0.426673 0.426673 0.426673 0.426673 0.426673 0.426673 0.466667 0.533333 0.559717 0.559717 0.559717 0.559717 0.559717 0.559717
  spline S38 degree 5 poles (-4.1414, -4.9789) (-4.1394, -4.9856) (-4.1323, -5.0091) (-4.1226, -5.0427) (-4.1136, -5.0765) (-4.1052, -5.1104) (-4.0989, -5.1377) (-4.0966, -5.1479) knots -0.559717 -0.559717 -0.559717 -0.559717 -0.559717 -0.559717 -0.533333 -0.466667 -0.426673 -0.426673 -0.426673 -0.426673 -0.426673 -0.426673
  spline S39 degree 5 poles (-4.0966, -5.1479) (-4.095, -5.1547) (-4.0897, -5.1787) (-4.0812, -5.2198) (-4.0705, -5.2785) (-4.0591, -5.3551) (-4.0494, -5.4432) (-4.0429, -5.5323) (-4.0401, -5.6044) (-4.0394, -5.6589) (-4.0395, -5.6954) (-4.0396, -5.7137) knots -0.426673 -0.426673 -0.426673 -0.426673 -0.426673 -0.426673 -0.4 -0.333333 -0.266667 -0.2 -0.133333 -0.066667 0 0 0 0 0 0
  arc A30 (-4.0396, -5.7137) -> (-5.7315, -7.9882) centre (-1.3148, -9.507) ccw
  arc A31 (-5.7315, -7.9882) -> (-5.5064, -8.3318) centre (2.1465, -3.0724) ccw
  arc A32 (-5.5064, -8.3318) -> (-2.7455, -7.6891) centre (-5.135, -3.6761) ccw
  spline S40 degree 5 poles (-2.7455, -7.6891) (-2.7286, -7.6962) (-2.6951, -7.7107) (-2.6454, -7.7332) (-2.5805, -7.7645) (-2.5014, -7.8061) (-2.4245, -7.8501) (-2.3588, -7.8911) (-2.3093, -7.9244) (-2.2749, -7.9486) (-2.2551, -7.9631) (-2.2495, -7.9672) knots 0 0 0 0 0 0 0.066667 0.133333 0.2 0.266667 0.333333 0.4 0.426673 0.426673 0.426673 0.426673 0.426673 0.426673
  spline S41 degree 5 poles (-2.2495, -7.9672) (-2.241, -7.9734) (-2.2185, -7.9901) (-2.1908, -8.0113) (-2.1634, -8.0331) (-2.1364, -8.0554) (-2.1177, -8.0713) (-2.1125, -8.0758) knots 0.426673 0.426673 0.426673 0.426673 0.426673 0.426673 0.466667 0.533333 0.559717 0.559717 0.559717 0.559717 0.559717 0.559717
  spline S42 degree 5 poles (-2.1125, -8.0758) (-2.1071, -8.0803) (-2.0885, -8.0962) (-2.0622, -8.1193) (-2.0363, -8.1428) (-2.0109, -8.1668) (-1.9909, -8.1863) (-1.9834, -8.1937) knots -0.559717 -0.559717 -0.559717 -0.559717 -0.559717 -0.559717 -0.533333 -0.466667 -0.426673 -0.426673 -0.426673 -0.426673 -0.426673 -0.426673
  spline S43 degree 5 poles (-1.9834, -8.1937) (-1.9784, -8.1986) (-1.961, -8.2159) (-1.9316, -8.2459) (-1.8908, -8.2895) (-1.8398, -8.3478) (-1.7841, -8.4166) (-1.7304, -8.4881) (-1.6891, -8.5472) (-1.659, -8.5926) (-1.6393, -8.6234) (-1.6296, -8.6389) knots -0.426673 -0.426673 -0.426673 -0.426673 -0.426673 -0.426673 -0.4 -0.333333 -0.266667 -0.2 -0.133333 -0.066667 0 0 0 0 0 0
  circle A33 centre (2.1465, -3.0724) radius 2.3876
  dimension "d5" = 4.7752
  constraint concentric A1 A33
  measures "d5" diameter of A33
extrude "Extrude2" cut sketch "Sketch3" against normal blind 12.7 contours A33
scale "Scale1" factor 0.9 about (-4.7728, 9.1045, 6.35) bodies 1